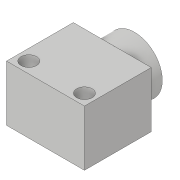
# Autodesk Inventor part: Part7
Saved by Autodesk Inventor 2017 (Build 210142000, 142)
## iProperties
Created: 2017-05-11
Part Number: Part7
Material: Generic
Document SubType Name: Modeling
Designer: zallen
Density: 1 g/cm^3
Appearance: Default
Author: zallen
Autodesk Inventor part; units mm, degrees
ref_plane "YZ Plane" through (0, 0, 0) normal (1, 0, 0) x (0, 1, 0)
ref_plane "XZ Plane" through (0, 0, 0) normal (0, 1, 0) x (-1, 0, 0)
ref_plane "XY Plane" through (0, 0, 0) normal (0, 0, 1) x (1, 0, 0)
sketch "Sketch1" plane through (0, 0, 0) normal (0, 0, 1) x (1, 0, 0)
  line L0 (-17.5, -12.5) -> (17.5, -12.5)
  line L1 (17.5, -12.5) -> (17.5, 12.5)
  line L2 (17.5, 12.5) -> (-17.5, 12.5)
  line L3 (-17.5, 12.5) -> (-17.5, -12.5)
  line L4 (-17.5, -12.5) -> (17.5, 12.5) construction
  line L5 (17.5, -12.5) -> (-17.5, 12.5) construction
  point P0 (0, 0)
  dimension "d0" = 35
  dimension "d1" = 25
  constraints: 12 end point, 2 midpoint, 2 parallel, 1 horizontal, 1 perpendicular
  measures "d0" distance of L2.end L1.end
  measures "d1" distance of L1.end L0.end
extrude "Extrusion1" add sketch "Sketch1" along normal blind 30
sketch "Sketch2" plane through (0, 0, 0) normal (0, 0, -1) x (-1, 0, 0)
  circle A0 centre (0, 0) radius 12.5
  dimension "d4" = 25
  constraints: 1 centre point, 1 coincident
  measures "d4" diameter of A0
extrude "Extrusion2" add sketch "Sketch2" along normal blind 10
sketch "Sketch3" plane through (-17.5, 12.5, 30) normal (0, 1, 0) x (1, 0, 0)
  circle A0 centre (30, 5) radius 3.5
  circle A1 centre (5, 5) radius 3.5
  line L0 (35, 0) -> (0, 0) projected
  line L1 (0, 30) -> (0, 0) projected
  line L2 (35, 30) -> (35, 0) projected
  point P0 (17.5, 30)
  dimension "d7" = 7
  dimension "d8" = 7
  dimension "d9" = 5
  dimension "d10" = 5
  dimension "d11" = 5
  dimension "d12" = 5
  constraints: 2 centre point
  measures "d7" diameter of A0
  measures "d8" diameter of A1
  measures "d9" distance from line of A1.centre L0
  measures "d10" distance from line of L1 A1.centre
  measures "d11" distance from line of L2 A0.centre
  measures "d12" distance from line of L0 A0.centre
extrude "Extrusion3" cut sketch "Sketch3" against normal through all
body "Solid1"
